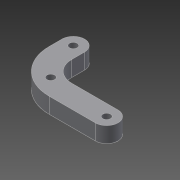
# Autodesk Inventor part: TEST
Saved by Autodesk Inventor 2014 SP1 (Build 180222100, 222)
## iProperties
Created: 2014-03-23
Part Number: TEST
Material: Generic
Document SubType Name: Modeling
Designer: Mark
Density: 1 g/cm^3
Appearance: Default
Author: Mark
Autodesk Inventor part; units mm, degrees
ref_plane "Right (YZ)" through (0, 0, 0) normal (1, 0, 0) x (0, 1, 0)
ref_plane "Top (XZ)" through (0, 0, 0) normal (0, 1, 0) x (-1, 0, 0)
ref_plane "Front (XY)" through (0, 0, 0) normal (0, 0, 1) x (1, 0, 0)
sketch "Sketch1" plane through (0, 0, 0) normal (0, 1, 0) x (-1, 0, 0)
  line L0 (0, 0) -> (11.3981, 0) construction
  line L1 (0, -2.2875) -> (9.3866, -2.2875)
  line L2 (9.3866, 2.2875) -> (0, 2.2875)
  arc A0 (0, 2.2875) -> (0, -2.2875) centre (0, 0) ccw
  arc A1 (18.1423, -6.4681) -> (9.3866, 2.2875) centre (9.3866, -6.4681) ccw
  arc A2 (13.5673, -6.4681) -> (9.3866, -2.2875) centre (9.3866, -6.4681) ccw
  line L3 (13.5673, -6.4681) -> (13.5673, -9.0771)
  arc A3 (13.5673, -9.0771) -> (18.1423, -9.0771) centre (15.8548, -9.0771) ccw
  line L4 (18.1423, -9.0771) -> (18.1423, -6.4681)
  point P0 (5.699, 0)
  constraints: 12 end point, 8 point on circle, 8 tangent, 4 centre point, 2 horizontal, 2 parallel, 1 concentric, 1 horizontal alignment, 1 midpoint, 1 perpendicular
extrude "Extrusion1" add sketch "Sketch1" against normal blind 3.175
hole "Hole1" at (-15.8548, 0, -9.0771) direction (0, -1, 0) diameter 1.5875 end through all
hole "Hole2" at (0, 0, 0) direction (0, -1, 0) diameter 1.5875 end through all
hole "Hole3" at (-12.5463, 0, -1.2005) direction (0, -1, 0) diameter 1.5875 end through all
equation "\"d13\" = d4"
equation "\"d4\" = 1.5875"
body "Solid1"
